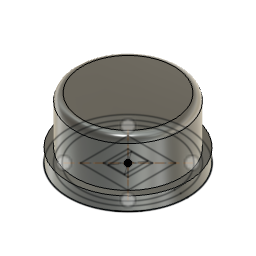
on_off_switch v6 (Autodesk Fusion 360 design; units mm, degrees)
Autodesk Fusion 360 part; units mm, degrees
sketch "Skizze1" plane through (0, 0, 0) normal (0, 0, 1) x (1, 0, 0)
  circle A0 centre (0, 0) radius 7.8
  circle A1 centre (0, 0) radius 8.8
  line L0 (1.2, -1.7) -> (-1.2, -1.7)
  line L1 (-1.2, -1.7) -> (-1.2, 1.7)
  line L2 (-1.2, 1.7) -> (1.2, 1.7)
  line L3 (1.2, 1.7) -> (1.2, -1.7)
  line L4 (1.2, -1.7) -> (-1.2, 1.7) construction
  line L5 (-1.2, -1.7) -> (1.2, 1.7) construction
  line L6 (4.75, -4.75) -> (-4.75, 4.75) construction
  line L7 (-4.75, -4.75) -> (4.75, 4.75) construction
  circle A2 centre (0, 0) radius 6.9
  line L8 (-1.8, -1.8) -> (1.8, -1.8)
  line L9 (1.8, -1.8) -> (1.8, 1.8)
  line L10 (1.8, 1.8) -> (-1.8, 1.8)
  line L11 (-1.8, 1.8) -> (-1.8, -1.8)
  line L12 (-1.8, -1.8) -> (1.8, 1.8) construction
  line L13 (1.8, -1.8) -> (-1.8, 1.8) construction
  line L14 (-3.5, -3.5) -> (3.5, -3.5)
  line L15 (3.5, -3.5) -> (3.5, 3.5)
  line L16 (3.5, 3.5) -> (-3.5, 3.5)
  line L17 (-3.5, 3.5) -> (-3.5, -3.5)
  line L18 (-3.5, -3.5) -> (3.5, 3.5) construction
  line L19 (3.5, -3.5) -> (-3.5, 3.5) construction
  dimension "d1" = 15.6
  dimension "d2" = 17.6
  dimension "d5" = 2.4
  dimension "d6" = 3.4
  dimension "d17" = 13.8
  dimension "d18" = 3.6
  dimension "d19" = 3.6
  dimension "d20" = 7
  dimension "d21" = 7
  constraint coincident A0.centre A1.centre
  constraint concentric A0 A1
  constraint horizontal L0
  constraint perpendicular L0 L1
  constraint parallel L0 L2
  constraint parallel L1 L3
  constraint coincident L4 A0.centre
  constraint coincident L5 A0.centre
  constraint coincident L6 A0.centre
  constraint coincident L7 A0.centre
  constraint horizontal L8
  constraint perpendicular L8 L9
  constraint parallel L8 L10
  constraint parallel L9 L11
  constraint coincident L12 A0.centre
  constraint coincident L13 A0.centre
  constraint horizontal L14
  constraint perpendicular L14 L15
  constraint parallel L14 L16
  constraint parallel L15 L17
  constraint coincident L18 A0.centre
  constraint coincident L19 A0.centre
  measures "d1" diameter of A0
  measures "d2" diameter of A1
  measures "d5" distance of L1 L3
  measures "d6" distance of L0 L2
  measures "d17" diameter of A2
  measures "d18" distance of L9 L11
  measures "d19" distance of L8 L10
  measures "d20" distance of L14 L16
  measures "d21" distance of L15 L17
extrude "Extrusion1" add sketch "Skizze1" along normal blind 9 contours A0 | L0 L1 L2 L3 | A2 | L8 L9 L10 L11 | L14 L15 L16 L17
extrude "Extrusion2" add sketch "Skizze1" along normal blind 2 contours A1
extrude "Extrusion5" cut sketch "Skizze1" along normal blind 8 contours A2
extrude "Extrusion6" cut sketch "Skizze1" along normal blind 5 contours L14 L15 L16 L17
extrude "Extrusion7" cut sketch "Skizze1" along normal blind 4.5 contours L8 L9 L10 L11
extrude "Extrusion8" cut sketch "Skizze1" along normal blind 7 contours L0 L1 L2 L3
fillet "Abrundung1" radius 1 1 edges at (-7.2722, -2.8206, 9)
